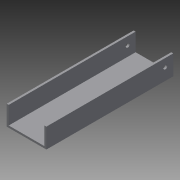
# Autodesk Inventor part: lower_leg
Saved by Autodesk Inventor 2015 (Build 190159000, 159)
## iProperties
Created: 2014-06-08
Part Number: lower_leg
Material: Generic
Document SubType Name: Modeling
Designer: L
Density: 1 g/cm^3
Appearance: Default
Author: L
Autodesk Inventor part; units mm, degrees
ref_plane "YZ Plane" through (0, 0, 0) normal (1, 0, 0) x (0, 1, 0)
ref_plane "XZ Plane" through (0, 0, 0) normal (0, 1, 0) x (-1, 0, 0)
ref_plane "XY Plane" through (0, 0, 0) normal (0, 0, 1) x (1, 0, 0)
sketch "Sketch1" plane through (0, 0, 0) normal (0, 0, 1) x (1, 0, 0)
  line L0 (0, 0) -> (127, 0)
  line L1 (127, 0) -> (127, 63.5)
  line L2 (127, 63.5) -> (120.65, 63.5)
  line L3 (120.65, 63.5) -> (120.65, 6.35)
  line L4 (120.65, 6.35) -> (6.35, 6.35)
  line L5 (6.35, 6.35) -> (6.35, 63.5)
  line L6 (6.35, 63.5) -> (0, 63.5)
  line L7 (0, 63.5) -> (0, 0)
  dimension "d0" = 127
  dimension "d1" = 63.5
  dimension "d2" = 6.35
  dimension "d3" = 57.15
  dimension "d4" = 114.3
  dimension "d5" = 57.15
  dimension "d6" = 6.35
  constraints: 16 end point, 4 perpendicular, 2 point on line, 1 horizontal
  measures "d0" distance of L0.start L0.end
  measures "d1" distance of L0.end L1.end
  measures "d2" distance of L1.end L2.end
  measures "d3" distance of L2.end L3.end
  measures "d4" distance of L3.end L4.end
  measures "d5" distance of L4.end L5.end
  measures "d6" distance of L5.end L6.end
extrude "Extrusion1" add sketch "Sketch1" along normal blind 406.4
sketch "Sketch2" plane through (127, 0, 0) normal (1, 0, 0) x (0, 0, -1)
  circle A0 centre (-25.4, 38.1) radius 6.35
  line L0 (0, 0) -> (0, 63.5) projected
  line L1 (0, 0) -> (-406.4, 0) projected
  dimension "d9" = 12.7
  dimension "d10" = 25.4
  dimension "d11" = 38.1
  constraints: 1 centre point
  measures "d9" diameter of A0
  measures "d10" distance from line of L0 A0.centre
  measures "d11" distance from line of L1 A0.centre
extrude "Extrusion2" cut sketch "Sketch2" against normal through all
equation "\"d0\" = o_width"
equation "\"d1\" = height"
equation "\"d2\" = thickness"
equation "\"d3\" = height - thickness"
equation "\"d4\" = i_width"
equation "\"d5\" = height - thickness"
equation "\"d6\" = thickness"
equation "\"d7\" = length"
equation "\"d9\" = mount_dia"
equation "\"d10\" = end_space"
equation "\"d11\" = mount_height"
equation "\"d12\" = length"
equation "\"o_width\" = 127"
equation "\"height\" = 0.5 * o_width"
equation "\"thickness\" = 6.35"
equation "\"i_width\" = o_width - 2 * thickness"
equation "\"length\" = 406.4"
equation "\"mount_dia\" = 12.7"
equation "\"mount_height\" = 38.1"
equation "\"end_space\" = 25.4"
body "Solid1"
